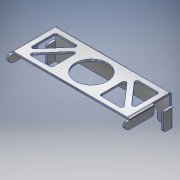
# Autodesk Inventor part: コックピット_サブフレーム_1_7
Saved by Autodesk Inventor 2018 (Build 220112000, 112)
## iProperties
Created: 2016-05-09
Part Number: コックピット_サブフレーム_1_7
Material: アルミニウム 5052
Document SubType Name: シート メタル
Designer: hiroaki
Density: 2.68 g/cm^3
Sheet Metal Rule: Default_mm
Appearance: アルミニウム - フラット
Mass: 32.2005 g
Surface Area: 139.179 cm^2
Volume: 12.0151 cm^3
Flat Pattern Width: 7.67109 cm
Flat Pattern Length: 13.3764 cm
Flat Pattern Area: 102.611 cm^2
Sheet Metal Width: 76.711 mm
Sheet Metal Length: 133.764 mm
Sheet Metal Area: 10261.143 mm^2
Author: hiroaki
Autodesk Inventor part; units mm, degrees
ref_plane "YZ Plane" through (0, 0, 0) normal (1, 0, 0) x (0, 1, 0)
ref_plane "XZ Plane" through (0, 0, 0) normal (0, 1, 0) x (-1, 0, 0)
ref_plane "XY Plane" through (0, 0, 0) normal (0, 0, 1) x (1, 0, 0)
sketch "スケッチ1" plane through (0, 0, 0) normal (0, 0, 1) x (1, 0, 0)
  line L0 (-59.5, -23.75) -> (59.5, -23.75)
  line L1 (59.5, -23.75) -> (59.5, 23.75)
  line L2 (59.5, 23.75) -> (-59.5, 23.75)
  line L3 (-59.5, 23.75) -> (-59.5, -23.75)
  line L4 (-59.5, -23.75) -> (59.5, 23.75) construction
  line L5 (59.5, -23.75) -> (-59.5, 23.75) construction
  point P0 (0, 0)
  dimension "d0" = 119
  dimension "d1" = 47.5
  constraints: 12 end point, 2 midpoint, 2 parallel, 1 horizontal, 1 perpendicular
  measures "d0" distance of L1.end L2.end
  measures "d1" distance of L2.end L0.start
extrude "押し出し1" add sketch "スケッチ1" along normal blind 2
sketch "スケッチ2" plane through (57.5, -23.75, 2) normal (1, 0, 0) x (0, 1, 0)
  line L0 (47.5, 0) -> (0, 0)
  line L1 (0, 0) -> (0, -10)
  line L2 (0, -10) -> (47.5, -10)
  line L3 (47.5, -10) -> (47.5, 0)
  constraints: 6 end point, 1 horizontal, 1 perpendicular, 1 vertical
edge flange "フランジ1" height 10 angle 90 thickness 2 bend radius 0.001 thickness toward (1, 0, 0) relief straight relief width 2 relief depth 1 corner gap 2 corner form 0 edges at (59.5, 0, 0) (-59.5, 0, 0) wall of the first edge with corners at (57.5, 23.75, 2) (57.5, -23.75, 2) (57.5, -23.75, -8) (57.5, 23.75, -8)
bend "曲げ1"
corner "コーナー1"
fillet "コーナーR1" radius 6 2 edges at (58.5, -23.75, -8) (-58.5, -23.75, -8)
sketch "スケッチ5" plane through (0, 0, 2) normal (0, 0, 1) x (1, 0, 0)
  line L0 (-57.499, 23.75) -> (-57.499, -23.75) projected
  line L1 (-57.499, -23.75) -> (57.499, -23.75) projected
  line L2 (57.499, -23.75) -> (57.499, 23.75) projected
  line L3 (-67.4934, 6.25) -> (-57.499, 6.25)
  line L4 (-57.499, 6.25) -> (-57.499, 39.8029)
  line L5 (-57.499, 39.8029) -> (-67.4934, 39.8029)
  line L6 (-67.4934, 39.8029) -> (-67.4934, 6.25)
  line L7 (66.0682, 34.2314) -> (57.499, 34.2314)
  line L8 (57.499, 34.2314) -> (57.499, 6.25)
  line L9 (57.499, 6.25) -> (66.0682, 6.25)
  line L10 (66.0682, 6.25) -> (66.0682, 34.2314)
  point P0 (0, 0)
  dimension "d24" = 30
  dimension "d25" = 30
  constraints: 16 end point, 4 parallel, 2 collinear, 2 horizontal, 2 perpendicular
  measures "d24" distance between parallel lines of L1 L3
  measures "d25" distance between parallel lines of L1 L9
extrude "押し出し2" cut sketch "スケッチ5" against normal blind 10
sketch "スケッチ6" plane through (57.499, 23.751, -0.001) normal (0, 1, 0) x (-1, 0, 0)
  line L0 (114.998, 0) -> (0, 0)
  line L1 (0, 0) -> (0, -27.999)
  line L2 (0, -27.999) -> (114.998, -27.999)
  line L3 (114.998, -27.999) -> (114.998, 0)
  constraints: 6 end point, 1 horizontal, 1 perpendicular, 1 vertical
edge flange "フランジ2" height 30 angle 90 thickness 2 bend radius 0.001 thickness toward (0, 1, 0) relief straight relief width 2 relief depth 1 edges at (0, 23.75, 0) wall of the first edge with corners at (-57.499, 23.751, -0.001) (57.499, 23.751, -0.001) (57.499, 23.751, -28) (-57.499, 23.751, -28)
bend "曲げ2"
corner "コーナー2"
sketch "スケッチ7" plane through (-57.5, 23.75, -28) normal (-1, 0, 0) x (0, -1, 0)
  line L0 (0, 27.999) -> (0, 0)
  line L1 (0, 0) -> (7.999, 0)
  line L2 (7.999, 0) -> (7.999, 27.999)
  line L3 (7.999, 27.999) -> (0, 27.999)
  constraints: 6 end point, 1 horizontal, 1 perpendicular, 1 vertical
edge flange "フランジ3" height 10 angle 90 thickness 2 bend radius 0.001 thickness toward (-1, 0, 0) relief straight relief width 2 relief depth 1 corner gap 2 corner form 0 edges at (-57.499, 23.751, -14.0005) (57.499, 23.751, -14.0005) wall of the first edge with corners at (-57.5, 23.75, -0.001) (-57.5, 23.75, -28) (-57.5, 15.751, -28) (-57.5, 15.751, -0.001)
bend "曲げ3"
corner "コーナー3"
sketch "スケッチ8" plane through (-57.499, 25.751, -0.001) normal (0, 1, 0) x (1, 0, 0)
  line L0 (0, 0) -> (114.998, 0) projected
  line L1 (114.998, 27.999) -> (114.998, 0) projected
  line L2 (0, 0) -> (0, 27.999) projected
  line L3 (124.0922, -5.5547) -> (114.998, -5.5547)
  line L4 (114.998, -5.5547) -> (114.998, 10)
  line L5 (114.998, 10) -> (124.0922, 10)
  line L6 (124.0922, 10) -> (124.0922, -5.5547)
  line L7 (-4.8753, -7.9113) -> (0, -7.9113)
  line L8 (0, -7.9113) -> (0, 10)
  line L9 (0, 10) -> (-4.8753, 10)
  line L10 (-4.8753, 10) -> (-4.8753, -7.9113)
  point P0 (57.499, -0.001)
  dimension "d48" = 10
  dimension "d49" = 10
  constraints: 16 end point, 4 parallel, 2 horizontal, 2 perpendicular, 1 collinear, 1 point on line
  measures "d48" distance between parallel lines of L0 L5
  measures "d49" distance between parallel lines of L9 L0
extrude "押し出し3" cut sketch "スケッチ8" against normal blind 10
sketch "スケッチ10" plane through (-57.499, 25.751, -28) normal (0, 1, 0) x (1, 0, 0)
  line L0 (0, 0) -> (114.998, 0) projected
  line L1 (102.499, 15.3147) -> (12.499, 15.3147)
  line L2 (12.499, 15.3147) -> (12.499, -10)
  line L3 (12.499, -10) -> (102.499, -10)
  line L4 (102.499, -10) -> (102.499, 15.3147)
  line L5 (57.499, -28) -> (57.499, 0) construction
  dimension "d63" = 10
  dimension "d64" = 90
  constraints: 10 end point, 2 parallel, 1 horizontal, 1 midpoint, 1 perpendicular, 1 other
  measures "d63" distance between parallel lines of L3 L0
  measures "d64" distance of L2.end L3.end
extrude "押し出し4" cut sketch "スケッチ10" against normal blind 10
fillet "フィレット1" radius 2 10 edges at (45, 24.751, -28) (45, 24.751, -18) (-45, 24.751, -18) (-45, 24.751, -28) (-58.5, 6.25, -8) (58.5, 6.25, -8) (-58.5, 15.751, -10.001) (58.5, 15.751, -10.001) (-58.5, 15.751, -28) (58.5, 15.751, -28)
sketch "スケッチ12" plane through (59.5, -23.75, -0.001) normal (1, 0, 0) x (0, 0, -1)
  line L0 (0, 30) -> (0, 0) projected
  line L1 (1.999, 0) -> (0, 0) projected
  line L2 (-11.3449, 5) -> (0, 5)
  line L3 (0, 5) -> (0, -9.2361)
  line L4 (0, -9.2361) -> (-11.3449, -9.2361)
  line L5 (-11.3449, -9.2361) -> (-11.3449, 5)
  point P0 (-0.001, 23.75)
  dimension "d71" = 5
  constraints: 8 end point, 2 parallel, 1 collinear, 1 horizontal, 1 perpendicular
  measures "d71" distance between parallel lines of L1 L2
extrude "押し出し6" cut sketch "スケッチ12" against normal blind 120
fillet "フィレット2" radius 3 2 edges at (58.5, -23.75, -0.001) (-58.5, -23.75, -0.001)
sketch "スケッチ15" plane through (0, 0, 2) normal (0, 0, 1) x (1, 0, 0)
  circle A0 centre (-20, 7.5) radius 0.7835 projected
  line L0 (-57.499, -18.75) -> (57.499, -18.75) projected
  line L1 (57.499, 23.75) -> (-57.499, 23.75) projected
  line L2 (-57.499, 6.25) -> (-57.499, -18.75) projected
  line L3 (-52.499, 18.75) -> (-52.499, -9.9582)
  line L4 (-52.499, -9.9582) -> (-27.325, 18.75)
  line L5 (-27.325, 18.75) -> (-52.499, 18.75)
  line L6 (-24, 14.9582) -> (-24, -13.75)
  line L7 (-24, -13.75) -> (-49.174, -13.75)
  line L8 (-49.174, -13.75) -> (-24, 14.9582)
  line L9 (-52.499, 18.75) -> (-24, 18.75) construction
  line L10 (-24, 18.75) -> (-24, -13.75) construction
  line L11 (-24, -13.75) -> (-52.499, -13.75) construction
  line L12 (-52.499, -13.75) -> (-52.499, 18.75) construction
  line L13 (-24, 18.75) -> (-52.499, -13.75) construction
  line L14 (-16, 18.75) -> (16, 18.75) construction
  line L15 (16, 18.75) -> (16, -13.75) construction
  line L16 (16, -13.75) -> (-16, -13.75) construction
  line L17 (-16, -13.75) -> (-16, 18.75) construction
  circle A1 centre (0, 2.5) radius 16.25
  line L18 (0, 0) -> (0, -18.75) construction
  line L19 (52.499, 18.75) -> (52.499, -9.9582)
  line L20 (52.499, -9.9582) -> (27.325, 18.75)
  line L21 (27.325, 18.75) -> (52.499, 18.75)
  line L22 (24, 14.9582) -> (24, -13.75)
  line L23 (24, -13.75) -> (49.174, -13.75)
  line L24 (49.174, -13.75) -> (24, 14.9582)
  line L25 (52.499, 18.75) -> (24, 18.75) construction
  line L26 (24, 18.75) -> (24, -13.75) construction
  line L27 (24, -13.75) -> (52.499, -13.75) construction
  line L28 (52.499, -13.75) -> (52.499, 18.75) construction
  line L29 (24, 18.75) -> (52.499, -13.75) construction
  point P0 (0, 18.75)
  dimension "d90" = 5
  dimension "d91" = 5
  dimension "d92" = 5
  dimension "d93" = 4
  dimension "d94" = 5
  dimension "d95" = 4
  constraints: 54 end point, 10 symmetric about line, 6 parallel, 4 collinear, 3 horizontal, 3 perpendicular, 2 horizontal alignment, 2 midpoint, 2 tangent, 2 vertical, 2 vertical alignment, 1 centre point, 1 other
  measures "d90" distance between parallel lines of L1 L9
  measures "d91" distance between parallel lines of L0 L11
  measures "d92" distance between parallel lines of L2 L12
  measures "d93" distance from line of A0.centre L10
  measures "d94" distance between parallel lines of L8 L4
  measures "d95" distance from line of L17 A0.centre
extrude "押し出し8" cut sketch "スケッチ15" against normal blind 10 contours L5 L4 L3 | L6 L7 L8 | A1 | L19 L20 L21 | L24 L23 L22
fillet "フィレット4" radius 2 12 edges at (-52.499, 18.75, 1) (-27.325, 18.75, 1) (-52.499, -9.9582, 1) (-49.174, -13.75, 1) (-24, 14.9582, 1) (27.325, 18.75, 1) (-24, -13.75, 1) (24, -13.75, 1) (52.499, -9.9582, 1) (49.174, -13.75, 1) (52.499, 18.75, 1) (24, 14.9582, 1)
equation "\"d25\" = d24"
equation "\"d49\" = d48"
equation "\"d91\" = d90"
equation "\"d92\" = d91"
equation "\"d95\" = d93"
equation "\"d4\" = BendReliefWidth"
equation "\"d5\" = BendReliefDepth"
equation "\"d6\" = MinimumRemnant"
equation "\"d7\" = BendRadius"
equation "\"d11\" = CornerReliefSize"
equation "\"d12\" = GapSize"
equation "\"d13\" = JacobiRadiusSize"
equation "\"d99\" = Thickness"
equation "\"d28\" = BendReliefWidth"
equation "\"d29\" = BendReliefDepth"
equation "\"d30\" = MinimumRemnant"
equation "\"d31\" = BendRadius"
equation "\"d35\" = CornerReliefSize"
equation "\"d36\" = GapSize"
equation "\"d37\" = JacobiRadiusSize"
equation "\"d38\" = BendReliefWidth"
equation "\"d39\" = BendReliefDepth"
equation "\"d40\" = MinimumRemnant"
equation "\"d41\" = BendRadius"
equation "\"d45\" = CornerReliefSize"
equation "\"d46\" = GapSize"
equation "\"d47\" = JacobiRadiusSize"
equation "\"BendRadius\" = Thickness"
equation "\"BendReliefWidth\" = Thickness"
equation "\"BendReliefDepth\" = 0.5 * Thickness"
equation "\"CornerReliefSize\" = 4 * Thickness"
equation "\"MinimumRemnant\" = 2 * Thickness"
equation "\"TransitionRadius\" = BendRadius"
equation "\"JacobiRadiusSize\" = BendRadius"
equation "\"GapSize\" = Thickness"
equation "\"Thickness\" = 2"
